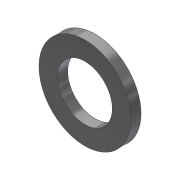
# Autodesk Inventor part: washer_nas620c2
Saved by Autodesk Inventor 2014 SP1 (Build 180222100, 222)
## iProperties
Created: 2020-06-23
Part Number: washer_nas620c2
Material: Stainless Steel
Document SubType Name: Modeling
Designer: RDavis
Density: 8.08 g/cm^3
Appearance: Semi-Polished
Author: RDavis
Autodesk Inventor part; units mm, degrees
ref_plane "YZ Plane" through (0, 0, 0) normal (1, 0, 0) x (0, 1, 0)
ref_plane "XZ Plane" through (0, 0, 0) normal (0, 1, 0) x (-1, 0, 0)
ref_plane "XY Plane" through (0, 0, 0) normal (0, 0, 1) x (1, 0, 0)
sketch "Sketch1" plane through (0, 0, 0) normal (0, 0, 1) x (1, 0, 0)
  circle A0 centre (0, 0) radius 1.1303
  circle A1 centre (0, 0) radius 1.8923
  dimension "d0" = 2.2606
  dimension "d1" = 3.7846
  constraints: 2 centre point, 2 coincident
  measures "d0" diameter of A0
  measures "d1" diameter of A1
extrude "Extrusion1" add sketch "Sketch1" along normal blind 0.4191
body "Solid1"
